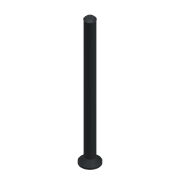
# Autodesk Inventor part: M3X40
Saved by Autodesk Inventor 2017 (Build 210142000, 142)
## iProperties
Part Number: M3X40
Material: Типовые
Document SubType Name: Modeling
Designer: STALKER
Density: 1 g/cm^3
Appearance: Чугун серый
Author: STALKER
Autodesk Inventor part; units mm, degrees
ref_plane "YZ Plane" through (0, 0, 0) normal (1, 0, 0) x (0, 1, 0)
ref_plane "XZ Plane" through (0, 0, 0) normal (0, 1, 0) x (-1, 0, 0)
ref_plane "XY Plane" through (0, 0, 0) normal (0, 0, 1) x (1, 0, 0)
sketch "Эскиз1" plane through (0, 0, 0) normal (0, 0, 1) x (1, 0, 0)
  circle A0 centre (0, 0) radius 1.5
  circle A1 centre (0, 0) radius 2.75
  line L0 (0, 1.1547) -> (1, 0.5774)
  line L1 (1, 0.5774) -> (1, -0.5774)
  line L2 (1, -0.5774) -> (0, -1.1547)
  line L3 (0, -1.1547) -> (-1, -0.5774)
  line L4 (-1, -0.5774) -> (-1, 0.5774)
  line L5 (-1, 0.5774) -> (0, 1.1547)
  dimension "d0" = 3
  dimension "d1" = 5.5
  dimension "d2" = 2
  constraints: 12 end point, 3 coincident, 2 centre point, 13 other
  measures "d0" diameter of A0
  measures "d1" diameter of A1
  measures "d2" distance between parallel lines of L1 L4
extrude "Выдавливание1" add sketch "Эскиз1" along normal blind 40 contours A0 | L0 L1 L2 L3 L4 L5
extrude "Выдавливание2" add sketch "Эскиз1" along normal blind 1.8 contours A1
chamfer "Фаска1" distance 1.25 angle 45 1 edges at (-2.75, 0, 1.8)
extrude "Выдавливание3" cut sketch "Эскиз1" along normal blind 1 contours L0 L1 L2 L3 L4 L5
chamfer "Фаска2" distance 0.5 angle 45 1 edges at (-1.5, 0, 40)
